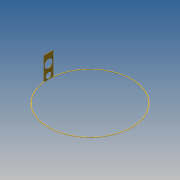
# Autodesk Inventor part: hubGuideRingOuter
Saved by Autodesk Inventor 2014 SP1 (Build 180222100, 222)
## iProperties
Created: 2014-12-05
Part Number: hubGuideRingOuter
Material: Gold
Document SubType Name: Modeling
Designer: Dave
Density: 19.3 g/cm^3
Appearance: Gold - Metal
Mass: 900.443 g
Surface Area: 514.308 cm^2
Volume: 46.6551 cm^3
Author: Dave
Autodesk Inventor part; units mm, degrees
ref_plane "YZ Plane" through (0, 0, 0) normal (1, 0, 0) x (0, 1, 0)
ref_plane "XZ Plane" through (0, 0, 0) normal (0, 1, 0) x (-1, 0, 0)
ref_plane "XY Plane" through (0, 0, 0) normal (0, 0, 1) x (1, 0, 0)
sketch "Sketch1" plane through (0, 0, 0) normal (0, 1, 0) x (-1, 0, 0)
  circle A0 centre (0, 0) radius 457.2
  circle A1 centre (0, 0) radius 463.55
  dimension "d0" = 914.4
  dimension "d1" = 6.35
  constraints: 2 centre point, 1 coincident
  measures "d0" diameter of A0
  measures "d1" radial gap between concentric circles of A0 A1
extrude "Extrusion1" add sketch "Sketch1" along normal blind 2.54
sketch "Sketch2" plane through (0, 2.54, 0) normal (0, 1, 0) x (1, 0, 0)
  line L0 (-459.74, -50.8) -> (-457.2, -50.8)
  line L1 (-457.2, -50.8) -> (-457.2, 50.8)
  line L2 (-457.2, 50.8) -> (-459.74, 50.8)
  line L3 (-459.74, 50.8) -> (-459.74, -50.8)
  line L4 (-459.74, 0) -> (-457.2, 0) construction
  dimension "d4" = 2.54
  dimension "d5" = 101.6
  constraints: 10 end point, 2 midpoint, 2 parallel, 2 perpendicular, 1 horizontal
  measures "d4" distance of L0.start L0.end
  measures "d5" distance of L0.end L1.end
extrude "Extrusion2" add sketch "Sketch2" along normal blind 254
sketch "Sketch3" plane through (0, 256.54, 0) normal (0, 1, 0) x (1, 0, 0)
  circle A0 centre (-458.47, 0) radius 0.254
  point P0 (0, 0)
  dimension "d8" = 0.508
  constraints: 1 centre point
  measures "d8" diameter of A0
extrude "Extrusion3" cut sketch "Sketch3" against normal blind 2.54
sketch "Sketch4" plane through (-459.74, 2.54, -50.8) normal (-1, 0, 0) x (0, 0, 1)
  line L0 (0, 254) -> (101.6, 254) projected
  circle A0 centre (50.8, 149.86) radius 45
  circle A1 centre (50.8, 35.5) radius 31.5
  point P0 (50.8, -2.54)
  dimension "d11" = 90
  dimension "d12" = 104.14
  dimension "d13" = 63
  dimension "d14" = 218.5
  constraints: 2 centre point
  measures "d11" diameter of A0
  measures "d12" distance from line of A0.centre L0
  measures "d13" diameter of A1
  measures "d14" distance from line of A1.centre L0
extrude "Extrusion4" cut sketch "Sketch4" against normal through all
equation "\"d0\" = hubOuterDiam"
equation "\"d11\" = sleeveOD"
equation "\"d13\" = sparOD"
equation "\"hubOuterDiam\" = 914.4"
equation "\"hubInnerDiam\" = 0.5 * hubOuterDiam"
equation "\"sleeveOD\" = 90"
equation "\"sparOD\" = 63"
body "Solid1"
